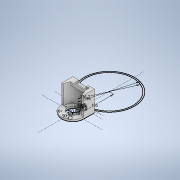
# Autodesk Inventor part: Cycloid_2_v1
Saved by Autodesk Inventor 2020.3 (Build 243373000, 373)
## iProperties
Created: 2021-04-18
Part Number: Cycloid_2_v1
Material: Generic
Document SubType Name: Modeling
Designer: sanyi
Density: 1 g/cm^3
Appearance: Default
Author: sanyi
Autodesk Inventor part; units mm, degrees
ref_plane "YZ Plane" through (0, 0, 0) normal (1, 0, 0) x (0, 1, 0)
ref_plane "XZ Plane" through (0, 0, 0) normal (0, 1, 0) x (-1, 0, 0)
ref_plane "XY Plane" through (0, 0, 0) normal (0, 0, 1) x (1, 0, 0)
sketch "Sketch1" plane through (0, 0, 0) normal (0, 1, 0) x (-1, 0, 0)
  circle A0 centre (0, 0) radius 15.25
  circle A1 centre (0, 0) radius 25 construction
  circle A2 centre (0, -105) radius 68.1
  line L0 (-85.4561, 0) -> (89.9732, 0) construction
  line L1 (0, 101.2907) -> (0, -205.3562) construction
  circle A3 centre (0, -105) radius 72
  line L2 (79.2949, -26.4) -> (-61.3617, -26.4) construction
  line L3 (49.9077, -36.9) -> (-43.2586, -36.9) construction
  circle A4 centre (0, 0) radius 31
  line L4 (31, 0) -> (31, -31.4)
  line L5 (-31, 0) -> (-31, -31.4)
  line L6 (31, -24.9) -> (-31, -24.9) construction
  line L7 (31, -21.3) -> (-31, -21.3)
  line L8 (31, -31.4) -> (-31, -31.4)
  circle A5 centre (3.65, -26.4) radius 1 construction
  circle A6 centre (10.15, -26.4) radius 1 construction
  circle A7 centre (-3.65, -26.4) radius 1 construction
  circle A8 centre (-10.15, -26.4) radius 1 construction
  line L9 (6.9, -21.3) -> (6.9, -31.4) construction
  line L10 (0.5, -21.3) -> (0.5, -31.4) construction
  line L11 (13.3, -21.3) -> (13.3, -31.4) construction
  line L12 (-6.9, -21.3) -> (-6.9, -31.4) construction
  line L13 (-0.5, -21.3) -> (-0.5, -31.4) construction
  line L14 (-13.3, -21.3) -> (-13.3, -31.4) construction
  line L15 (32.3583, -36.4) -> (-52.2752, -36.4) construction
  line L16 (31.0245, -33.2) -> (-40.7882, -33.2) construction
  line L17 (0, 0) -> (20, 0)
  line L18 (0, 0) -> (-10, 17.3205)
  line L19 (0, 0) -> (-10, -17.3205)
  line L20 (0, 17.3205) -> (-18.0278, 17.3205) construction
  line L21 (0, -17.3205) -> (-18.0278, -17.3205) construction
  circle A9 centre (-10, 17.3205) radius 2.1
  circle A10 centre (20, 0) radius 2.1
  circle A11 centre (-10, -17.3205) radius 2.1
  dimension "d0" = 30.5
  dimension "d1" = 50
  dimension "d2" = 136.2
  dimension "d3" = 105
  dimension "d4" = 144
  dimension "d5" = 10.5
  dimension "d6" = 6
  dimension "d7" = 1.5
  dimension "d8" = 3.6
  dimension "d10" = 6.5
  dimension "d12" = 2
  dimension "d14" = 6.5
  dimension "d15" = 6.5
  dimension "d16" = 12.8
  dimension "d17" = 12.8
  dimension "d18" = 1
  dimension "d19" = 10
  dimension "d20" = 6.8
  dimension "d21" = 120
  dimension "d22" = 120
  dimension "d23" = 20
  dimension "d24" = 4.2
  constraints: 46 end point, 29 point on line, 12 centre point, 9 perpendicular, 7 coincident, 6 horizontal, 6 parallel, 5 equal radius, 4 point on circle, 3 tangent, 3 vertical, 2 equal length, 2 symmetric about line, 1 collinear, 3 other
  measures "d0" diameter of A0
  measures "d1" diameter of A1
  measures "d2" diameter of A2
  measures "d3" distance of point (0, 0) A2.centre
  measures "d4" diameter of A3
  measures "d5" distance between parallel lines of L2 L3
  measures "d6" radial gap between concentric circles of A4 A1
  measures "d7" distance between parallel lines of L2 L6
  measures "d8" distance between parallel lines of L7 L6
  measures "d10" distance between parallel lines of L6 L8
  measures "d12" diameter of A6
  measures "d14" distance of A5.centre A6.centre
  measures "d15" distance of A8.centre A7.centre
  measures "d16" distance between parallel lines of L10 L11
  measures "d17" distance between parallel lines of L14 L13
  measures "d18" distance between parallel lines of L10 L13
  measures "d19" distance between parallel lines of L15 L2
  measures "d20" distance between parallel lines of L2 L16
  measures "d21" angle of L19 L17
  measures "d22" angle of L18 L19
  measures "d23" distance of L17.start L19.end
  measures "d24" diameter of A9
extrude "Extrusion1" add sketch "Sketch1" along normal blind 5 contours A4 L7 | L4 L7 A4 | A4 L7 L5 | L7 L4 L8 L5 A4 | A4 L7
sketch "Sketch2" plane through (0, 5, 0) normal (0, 1, 0) x (1, 0, 0)
  arc A0 (-31, 0) -> (31, 0) centre (0, 0) ccw projected
  line L0 (31, 0) -> (31, 31.4) projected
  line L1 (31, 31.4) -> (-31, 31.4) projected
  line L2 (-31, 31.4) -> (-31, 0) projected
  circle A1 centre (-20, 0) radius 2.1 projected
  circle A2 centre (10, -17.3205) radius 2.1 projected
  circle A3 centre (0, 0) radius 15.25 projected
  circle A4 centre (10, 17.3205) radius 2.1 projected
  circle A5 centre (0, 0) radius 25 construction
  circle A6 centre (0, 0) radius 26
  line L3 (31, 0) -> (31, 31.4) projected
  line L4 (26, 0) -> (31, 0)
  arc A7 (-31, 0) -> (31, 0) centre (0, 0) ccw projected
  line L5 (-26, 0) -> (-31, 0)
  line L6 (-7.5, 26) -> (7.5, 26) construction
  line L7 (0, -101.2907) -> (0, 205.3562) construction
  line L8 (0, 0) -> (-20, 0) projected
  line L9 (31, 31.4) -> (-31, 31.4) projected
  line L10 (-7.5, 24.8948) -> (-7.5, 31.4)
  line L11 (7.5, 24.8948) -> (7.5, 31.4)
  line L12 (-79.2949, 26.4) -> (61.3617, 26.4) construction
  circle A8 centre (19.25, 24.9) radius 2.5
  line L13 (19.25, 21.3141) -> (19.25, 28.7892) construction
  line L14 (17.25, 26.4) -> (21.25, 26.4)
  line L15 (-31, 24.9) -> (31, 24.9) construction
  dimension "d27" = 1
  dimension "d28" = 15
  dimension "d37" = 5
  constraints: 14 end point, 8 point on line, 6 point on circle, 4 perpendicular, 2 centre point, 2 horizontal, 1 coincident, 1 symmetric about line, 1 tangent, 1 other
  measures "d27" radial gap between concentric circles of A6 A5
  measures "d28" distance of L6.start L6.end
  measures "d37" diameter of A8
extrude "Extrusion2" add sketch "Sketch2" along normal blind 20 contours L2 L1 L10 A6 L5 | L4 A6 L11 L1 L0
sketch "Sketch3" plane through (0, 25, 0) normal (0, 1, 0) x (1, 0, 0)
  line L0 (-31, 0) -> (-26, 0) projected
  arc A0 (-7.5, 24.8948) -> (-26, 0) centre (0, 0) ccw projected
  line L1 (-7.5, 24.8948) -> (-7.5, 31.4) projected
  line L2 (-7.5, 31.4) -> (-31, 31.4) projected
  line L3 (-31, 31.4) -> (-31, 0) projected
  line L4 (31, 0) -> (31, 31.4) projected
  line L5 (31, 31.4) -> (7.5, 31.4) projected
  line L6 (7.5, 31.4) -> (7.5, 24.8948) projected
  arc A1 (26, 0) -> (7.5, 24.8948) centre (0, 0) ccw projected
  line L7 (26, 0) -> (31, 0) projected
  circle A2 centre (0, 0) radius 26 projected
  line L8 (7.5, 31.4) -> (-7.5, 31.4) projected
  circle A3 centre (19.25, 24.9) radius 2.5 projected
extrude "Extrusion3" add sketch "Sketch3" along normal blind 25 contours L3 L2 L1 A0 L0 | L1 L8 L6 A2 | A1 L6 L5 L4 L7
full round fillet "Fillet1" first side at (7.5, 18.3333, -29.2316) centre faces at (0.844, 25, -29.5588) second side at (-7.5, 11.6667, -27.0632)
sketch "Sketch4" plane through (0, 50, 0) normal (0, 1, 0) x (1, 0, 0)
  line L0 (-31, 21.3) -> (31, 21.3) projected
  circle A0 centre (0, 0) radius 15.25 projected
  line L1 (-31, 0) -> (-26, 0) projected
  arc A1 (26, 0) -> (-26, 0) centre (0, 0) ccw projected
  line L2 (26, 0) -> (31, 0) projected
  line L3 (31, 0) -> (31, 31.4) projected
  line L4 (31, 31.4) -> (-31, 31.4) projected
  line L5 (-31, 31.4) -> (-31, 0) projected
  line L6 (-31, 15.25) -> (31, 15.25)
  line L7 (-31, 31.4) -> (-31, 0) projected
  circle A2 centre (19.25, 24.9) radius 2.5 projected
  point P0 (21.058, 15.25)
  point P1 (-21.058, 15.25)
  constraints: 2 end point, 2 point on line, 1 perpendicular, 1 tangent
extrude "Extrusion4" add sketch "Sketch4" along normal blind 3 contours L5 L4 L3 L0 A1 | L0 A1 L6 L5 | A1 L0 | L0 A1 L6 | L6 A1 L1 L5 | L0 L3 L6 A1 | L6 L3 L2 A1
sketch "Sketch5" plane through (0, 53, 0) normal (0, 1, 0) x (1, 0, 0)
  line L0 (-31, 21.3) -> (31, 21.3) projected
  line L1 (26, 0) -> (31, 0) projected
  line L2 (31, 0) -> (31, 31.4) projected
  line L3 (31, 31.4) -> (-31, 31.4) projected
  line L4 (-31, 31.4) -> (-31, 0) projected
  line L5 (-31, 0) -> (-26, 0) projected
  arc A0 (-21.058, 15.25) -> (-26, 0) centre (0, 0) ccw projected
  line L6 (-21.058, 15.25) -> (21.058, 15.25) projected
  arc A1 (26, 0) -> (21.058, 15.25) centre (0, 0) ccw projected
  line L7 (13.3, 21.3) -> (13.3, 31.4) projected
  circle A2 centre (10.15, 26.4) radius 1 construction
  circle A3 centre (3.65, 26.4) radius 1 construction
  line L8 (0.5, 21.3) -> (0.5, 31.4) construction
  line L9 (-0.5, 21.3) -> (-0.5, 31.4) construction
  circle A4 centre (-3.65, 26.4) radius 1 construction
  circle A5 centre (-10.15, 26.4) radius 1 construction
  line L10 (-13.3, 21.3) -> (-13.3, 31.4) projected
  arc A6 (21.058, 15.25) -> (-21.058, 15.25) centre (0, 0) ccw construction
  circle A7 centre (10.15, 26.4) radius 0.8
  circle A8 centre (3.65, 26.4) radius 0.8
  circle A9 centre (-3.65, 26.4) radius 0.8
  circle A10 centre (-10.15, 26.4) radius 0.8
  line L11 (-18.5186, 18.25) -> (18.5186, 18.25)
  line L12 (-21.058, 15.25) -> (21.058, 15.25) projected
  line L13 (-31, 24.9) -> (31, 24.9) construction
  circle A11 centre (19.25, 24.9) radius 2.5 projected
  line L14 (13.3, 24.9) -> (16.75, 24.9)
  line L15 (18.5186, 18.25) -> (21.058, 18.25)
  line L16 (21.058, 18.25) -> (21.736, 24.636)
  arc A12 (26, 0) -> (21.058, 15.25) centre (0, 0) ccw projected
  line L17 (21.058, 15.25) -> (21.058, 23.1734) construction
  line L18 (-13.3, 21.3) -> (-13.3, 18.25)
  dimension "d35" = 1.6
  dimension "d36" = 3
  constraints: 12 end point, 6 point on line, 5 point on circle, 4 centre point, 4 coincident, 3 equal radius, 2 vertical, 1 parallel, 1 tangent
  measures "d35" diameter of A7
  measures "d36" distance between parallel lines of L6 L11
extrude "Extrusion5" add sketch "Sketch5" along normal blind 5.8 contours L4 L3 L10 L0 | L0 L18 L11 L15 L16 L2 L1 A1 L6 A0 L5 L4 | L16 A11 L14 L7 L3 L2 L0
body "Solid1"
